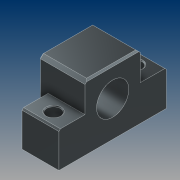
# Autodesk Inventor part: Goi_do_B
Saved by Autodesk Inventor 2021 (Build 250183000, 183)
## iProperties
Created: 2024-04-08
Part Number: Goi_do_B
Material: Iron, Gray
Document SubType Name: Modeling
Designer: Admin
Density: 7.15 g/cm^3
Appearance: Iron Gray
Author: Admin
Autodesk Inventor part; units mm, degrees
ref_plane "YZ Plane" through (0, 0, 0) normal (1, 0, 0) x (0, 1, 0)
ref_plane "XZ Plane" through (0, 0, 0) normal (0, 1, 0) x (-1, 0, 0)
ref_plane "XY Plane" through (0, 0, 0) normal (0, 0, 1) x (1, 0, 0)
sketch "Sketch1" plane through (0, 0, 0) normal (1, 0, 0) x (0, 1, 0)
  line L0 (-24, 35) -> (24, 35)
  line L1 (24, 35) -> (24, -35)
  line L2 (24, -35) -> (-24, -35)
  line L3 (-24, -35) -> (-24, 35)
  line L4 (-24, 35) -> (24, -35) construction
  line L5 (24, 35) -> (-24, -35) construction
  line L6 (-43, 18) -> (43, 18)
  line L7 (43, 18) -> (43, -18)
  line L8 (43, -18) -> (-43, -18)
  line L9 (-43, -18) -> (-43, 18)
  line L10 (-43, 18) -> (43, -18) construction
  line L11 (43, 18) -> (-43, -18) construction
  circle A0 centre (24, 0) radius 10.5
  line L12 (0, 35) -> (0, -35)
  point P0 (0, 0)
  point P1 (24, -18)
  point P2 (24, 18)
  dimension "d0" = 36
  dimension "d1" = 70
  dimension "d2" = 19
  dimension "d3" = 24
  dimension "d4" = 21
  constraints: 26 end point, 7 midpoint, 4 parallel, 2 horizontal, 2 perpendicular, 1 centre point
  measures "d0" distance between parallel lines of L6 L8
  measures "d1" distance between parallel lines of L0 L2
  measures "d2" distance between parallel lines of L7 L1
  measures "d3" distance from line of point (0, 0) L1
  measures "d4" diameter of A0
extrude "Extrusion1" add sketch "Sketch1" along normal mid plane 24 contours L0 L1 L6 L12 | L6 L1 A0 L8 L12 | L6 L7 L8 L1 A0 | L8 L1 L2 L12
sketch "Sketch2" plane through (-12, 24, -18) normal (0, 1, 0) x (1, 0, 0)
  line L0 (0, 0) -> (24, 0) projected
  line L1 (24, 17) -> (24, 0) projected
  line L2 (0, 17) -> (24, 17) projected
  line L3 (0, 0) -> (0, 17) projected
  line L4 (0, -53) -> (24, -53) projected
  line L5 (24, -36) -> (24, -53) projected
  line L6 (0, -36) -> (24, -36) projected
  line L7 (0, -53) -> (0, -36) projected
  line L8 (0, -53) -> (24, -36)
  line L9 (24, 17) -> (24, 0) projected
  line L10 (24, 0) -> (0, 17)
  point P0 (12, -18)
  point P1 (12, -44.5)
  point P2 (12, 8.5)
  constraints: 4 end point, 2 midpoint
hole "Hole1" at (0, 24, 26.5) at (0, 24, -26.5) direction (0, -1, 0) diameter 9 end through all
chamfer "Chamfer1" distance 1 angle 45 1 edges at (12, 43, 0)
chamfer "Chamfer2" distance 1 angle 45 6 edges at (0, 24, 35) (0, 24, -35) (-12, 0, 0) (0, 0, -35) (12, 0, 0) (0, 0, 35)
chamfer "Chamfer3" distance 2 angle 45 2 edges at (-0.5, 43, -18) (-0.5, 43, 18)
sketch "Sketch3" plane through (-12, 0, 0) normal (-1, 0, 0) x (0, 0, 1)
  line L0 (16, 43) -> (18, 41) projected
  line L1 (16, 43) -> (-16, 43) projected
  line L2 (-18, 41) -> (-16, 43) projected
  line L3 (-18, 41) -> (-18, 24) projected
  line L4 (-18, 24) -> (-34, 24) projected
  line L5 (-35, 23) -> (-34, 24) projected
  line L6 (-35, 23) -> (-35, 1) projected
  line L7 (35, 1) -> (-35, 1) projected
  line L8 (35, 1) -> (35, 23) projected
  line L9 (34, 24) -> (35, 23) projected
  line L10 (34, 24) -> (18, 24) projected
  line L11 (18, 24) -> (18, 41) projected
  circle A0 centre (0, 24) radius 10.5 projected
  line L12 (18, 5) -> (-18, 5)
  line L13 (-18, 5) -> (-18, 43)
  line L14 (-18, 43) -> (18, 43)
  line L15 (18, 43) -> (18, 5)
  line L16 (18, 5) -> (-18, 43) construction
  line L17 (-18, 5) -> (18, 43) construction
  line L18 (-14, 9) -> (14, 9)
  line L19 (14, 9) -> (14, 39)
  line L20 (14, 39) -> (-14, 39)
  line L21 (-14, 39) -> (-14, 9)
  point P0 (0, 0)
  dimension "d23" = 30
  constraints: 20 end point, 4 parallel, 2 midpoint, 2 perpendicular, 1 horizontal, 1 horizontal alignment, 1 vertical alignment, 3 other
  measures "d23" distance of L20.end L18.start
extrude "Extrusion2" add sketch "Sketch3" along normal blind 5.5 contours L0 L11 L15 L12 L13 L3 L2 L1 | L21 L20 L19 L18
sketch "Sketch4" plane through (-17.5, 0, 0) normal (-1, 0, 0) x (0, 0, 1)
  line L0 (18, 5) -> (18, 41) projected
  line L1 (18, 41) -> (16, 43) projected
  line L2 (16, 43) -> (-16, 43) projected
  line L3 (-16, 43) -> (-18, 41) projected
  line L4 (-18, 41) -> (-18, 5) projected
  line L5 (-18, 5) -> (18, 5) projected
  circle A0 centre (0, 24) radius 10.5 projected
  line L6 (14, 9) -> (14, 39)
  line L7 (14, 39) -> (-14, 39)
  line L8 (-14, 39) -> (-14, 9)
  line L9 (-14, 9) -> (14, 9)
  point P0 (0, 0)
  dimension "d26" = 4
  constraints: 8 end point, 3 other
  measures "d26" distance between parallel lines of L4 L8
hole "Hole2" at (-17.5, 9, 14) at (-17.5, 9, -14) at (-17.5, 39, -14) at (-17.5, 39, 14) direction (1, 0, 0) diameter 4 depth 5.5 tip angle 118 counterbore diameter 6 counterbore depth 2
chamfer "Chamfer4" distance 2 angle 45 2 edges at (-14.75, 5, 18) (-14.75, 5, -18)
chamfer "Chamfer5" distance 0.5 angle 45 8 edges at (-17.5, 43, 0) (-17.5, 42, 17) (-17.5, 24, 18) (-17.5, 24, -18) (-17.5, 42, -17) (-17.5, 6, -17) (-17.5, 5, 0) (-17.5, 6, 17)
chamfer "Chamfer6" distance 0.5 angle 45 2 edges at (0, 24, -31) (0, 24, 22)
body "Solid1"
